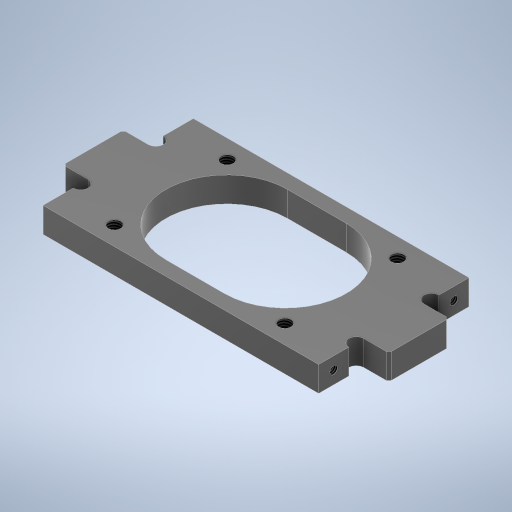
# Autodesk Inventor part: HeadSpeakerMountFrame
Saved by Autodesk Inventor 2024.2 (Build 282272000, 272)
## iProperties
Created: 2024-01-19
Part Number: HeadSpeakerMountFrame
Material: Acetal Resin, Black
Document SubType Name: Modeling
Designer: Masato Kubotera
Density: 1.425 g/cm^3
Appearance: Smooth - Black
Mass: 6.97229 g
Surface Area: 37.3223 cm^2
Volume: 4.89284 cm^3
Vendor: meviy
Author: Masato Kubotera
Autodesk Inventor part; units mm, degrees
ref_plane "YZ Plane" through (0, 0, 0) normal (1, 0, 0) x (0, 1, 0)
ref_plane "XZ Plane" through (0, 0, 0) normal (0, 1, 0) x (-1, 0, 0)
ref_plane "XY Plane" through (0, 0, 0) normal (0, 0, 1) x (1, 0, 0)
sketch "Sketch1" plane through (0, 0, 0) normal (0, 0, 1) x (1, 0, 0)
  line L0 (15, 27.5) -> (-15, 27.5)
  line L1 (-15, 27.5) -> (-15, -27.5)
  line L2 (-15, -27.5) -> (15, -27.5)
  line L3 (15, -27.5) -> (15, 27.5)
  line L4 (15, 27.5) -> (-15, -27.5) construction
  line L5 (-15, 27.5) -> (15, -27.5) construction
  line L6 (11.25, 17) -> (-11.25, 17) construction
  line L7 (-11.25, 17) -> (-11.25, -17) construction
  line L8 (-11.25, -17) -> (11.25, -17) construction
  line L9 (11.25, -17) -> (11.25, 17) construction
  line L10 (11.25, 17) -> (-11.25, -17) construction
  line L11 (-11.25, 17) -> (11.25, -17) construction
  line L12 (0, 27.5) -> (0, -27.5) construction
  line L13 (15, 0) -> (-15, 0) construction
  line L14 (6, 27.5) -> (6, 32.5)
  line L15 (6, 32.5) -> (-6, 32.5)
  line L16 (-6, 32.5) -> (-6, 27.5)
  arc A0 (-9, 27.5) -> (-6, 27.5) centre (-7.5, 27.5) ccw
  line L17 (6, -27.5) -> (6, -32.5)
  line L18 (6, -32.5) -> (-6, -32.5)
  line L19 (-6, -32.5) -> (-6, -27.5)
  arc A1 (-6, -27.5) -> (-9, -27.5) centre (-7.5, -27.5) ccw
  line L20 (-12, 27.5) -> (-12, 21.5) construction
  line L21 (0, 32.5) -> (0, 27.5) construction
  line L22 (12, 27.5) -> (12, 21.5) construction
  arc A2 (6, 27.5) -> (9, 27.5) centre (7.5, 27.5) ccw
  line L23 (12, -27.5) -> (12, -21.5) construction
  arc A3 (9, -27.5) -> (6, -27.5) centre (7.5, -27.5) ccw
  line L24 (-14.15, -20) -> (14.15, -20) construction
  line L25 (14.15, -20) -> (14.15, 20) construction
  line L26 (14.15, 20) -> (-14.15, 20) construction
  line L27 (-14.15, 20) -> (-14.15, -20) construction
  line L28 (-14.15, -20) -> (14.15, 20) construction
  line L29 (14.15, -20) -> (-14.15, 20) construction
  arc A4 (-12.15, -5.85) -> (12.15, -5.85) centre (0, -5.85) ccw
  line L30 (12.15, -5.85) -> (-12.15, -5.85) construction
  arc A5 (12.15, 5.85) -> (-12.15, 5.85) centre (0, 5.85) ccw
  line L31 (-12.15, -5.85) -> (-12.15, 5.85)
  line L32 (12.15, 5.85) -> (12.15, -5.85)
  circle A6 centre (11.25, 17) radius 1.5 construction
  point P0 (0, 0)
  point P1 (0, 0)
  point P2 (0, 0)
  point P3 (-9, -27.5)
  point P4 (6, -27.5)
  point P5 (-6, -27.5)
  point P6 (-6, -27.5)
  point P7 (6, -27.5)
  point P8 (9, -27.5)
  dimension "d0" = 22.5
  dimension "d1" = 34
  dimension "d19" = 5
  dimension "d37" = 55
  dimension "d40" = 6
  dimension "d41" = 6
  dimension "d57" = 30
  dimension "d58" = 1.5
  dimension "d59" = 28.3
  dimension "d60" = 40
  dimension "d61" = 2
  dimension "d62" = 2
  dimension "d63" = 9
  dimension "d64" = 12
  dimension "d65" = 3
  constraints: 65 end point, 16 symmetric about line, 14 midpoint, 12 point on circle, 7 centre point, 6 parallel, 5 vertical, 4 coincident, 4 horizontal, 2 perpendicular, 1 collinear, 1 point on line, 1 tangent, 16 other
  measures "d0" distance of L8.end L7.end
  measures "d1" distance of L7.end L6.end
  measures "d19" distance of L14.start L14.end
  measures "d37" distance of L2.end L3.end
  measures "d40" distance of L20.start L20.end
  measures "d41" distance between parallel lines of L16 L20
  measures "d57" distance between parallel lines of L1 L3
  measures "d58" radius of A2
  measures "d59" distance of L26.end L25.end
  measures "d60" distance of L25.end L24.end
  measures "d61" distance edge to line of A4 L24
  measures "d62" distance edge to line of A4 L25
  measures "d63" distance between parallel lines of L1 L16
  measures "d64" distance between parallel lines of L16 L14
  measures "d65" diameter of A6
extrude "Extrusion1" add sketch "Sketch1" against normal blind 5 contours L3 L2 A3 A1 L1 L0 A0 A2 | L0 L16 L15 L14 | L17 L18 L19 L2 | L31 A5 L32 A4
hole "Hole1" at (11.25, 17, 0) at (-11.25, 17, 0) at (-11.25, -17, 0) at (11.25, -17, 0) direction (0, 0, -1) diameter 2.459 end through all thread size "M3x0.5" class "6H" standard "ANSI Metric M Profile"
extrude "Extrusion2" cut sketch "Sketch1" against normal through all contours L31 A5 L32 A4
sketch "Sketch2" plane through (-15, 27.5, 0) normal (0, 1, 0) x (1, 0, 0)
  line L0 (3, 5) -> (3, 0)
  line L1 (30, 0) -> (0, 0) projected
  line L2 (27, 5) -> (27, 0)
  line L3 (24, 5) -> (30, 5) projected
  line L4 (0, 5) -> (6, 5) projected
  point P0 (15, 0)
  point P1 (6, 0)
  point P2 (3, 2.5)
  point P3 (3, 0)
  point P4 (27, 2.5)
  constraints: 4 end point, 4 midpoint, 2 vertical, 1 other
hole "Hole2" at (-12, 27.5, -2.5) at (12, 27.5, -2.5) direction (0, -1, 0) diameter 1.567 depth 6.3 thread size "M2x0.4" class "6H" standard "ANSI Metric M Profile"
mirror "Mirror1" about plane through (0, 0, 0) normal (0, 1, 0) of "Hole2"
chamfer "Chamfer1" distance 0.5 angle 45 4 edges at (6, -32.5, -2.5) (-6, -32.5, -2.5) (6, 32.5, -2.5) (-6, 32.5, -2.5)
body "Solid1"
